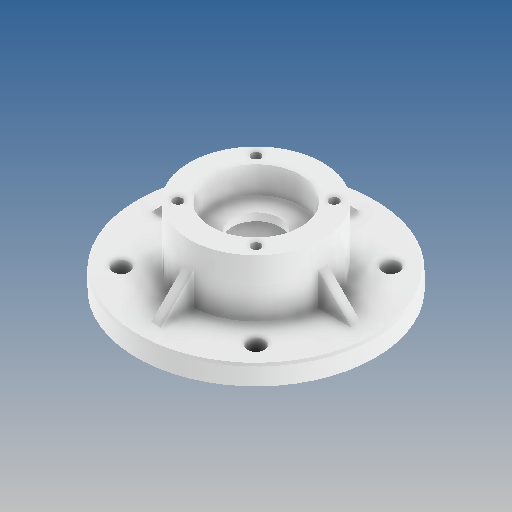
# Autodesk Inventor part: PWTR-0046
Saved by Autodesk Inventor 2021.1 (Build 251245000, 245)
## iProperties
Created: 2020-08-27
Part Number: PWTR-0046
Material: Aluminum 6061
Document SubType Name: Modeling
Designer: alid
Density: 2.7 g/cm^3
Appearance: Aluminum - Flat
Description: Transfer Case Connecting Plate
Author: alid
Revision Number: A
Autodesk Inventor part; units mm, degrees
ref_plane "YZ Plane" through (0, 0, 0) normal (1, 0, 0) x (0, 1, 0)
ref_plane "XZ Plane" through (0, 0, 0) normal (0, 1, 0) x (-1, 0, 0)
ref_plane "XY Plane" through (0, 0, 0) normal (0, 0, 1) x (1, 0, 0)
sketch "Sketch1" plane through (0, 0, 0) normal (0, 1, 0) x (-1, 0, 0)
  line L0 (0, 0) -> (0, 40)
  line L1 (0, 40) -> (-35, 40)
  line L2 (-35, 40) -> (-35, 10)
  line L3 (-35, 10) -> (-62.5, 10)
  line L4 (-62.5, 10) -> (-62.5, 0)
  line L5 (-62.5, 0) -> (0, 0)
  line L6 (-51.5, 11) -> (-36, 26.5)
  line L7 (-36, 40) -> (-36, 11) construction
  line L8 (-36, 11) -> (-72.5, 11) construction
  line L9 (-51.5, 11) -> (-52.5, 10) construction
  line L10 (0, 0) -> (0, -10)
  line L11 (0, -10) -> (-37.5, -10)
  line L12 (-37.5, -10) -> (-37.5, 0)
  dimension "d0" = 40
  dimension "d1" = 125
  dimension "d2" = 70
  dimension "d3" = 10
  dimension "d4" = 45
  dimension "d14" = 1
  dimension "d15" = 1
  dimension "d16" = 10
  dimension "d26" = 10
  dimension "d27" = 75
  constraints: 26 end point, 8 perpendicular, 4 point on line, 2 vertical, 1 collinear, 1 horizontal alignment, 1 parallel
  measures "d0" distance of L0.start L0.end
  measures "d1" diameter of L4 L0
  measures "d2" diameter of L2 L0
  measures "d3" distance between parallel lines of L5 L3
  measures "d4" angle of L3 L6
  measures "d14" distance between parallel lines of L3 L8
  measures "d15" distance between parallel lines of L2 L7
  measures "d16" distance from line of L4 L9.end
  measures "d26" distance of L0.start L10.end
  measures "d27" diameter of L12 L0
revolve "Revolution1" add sketch "Sketch1" angle 360 about axis through (0, 0, 0) along (0, 0, 1)
extrude "Rib1" add sketch "Sketch1" along normal mid plane 5 rib yes fills toward (-43.7146, 18.7146) open curves L6
sketch "Sketch3" plane through (0, 0, 40) normal (0, 0, 1) x (1, 0, 0)
  circle A0 centre (0, 0) radius 35 projected
  constraints: 1 coincident
hole "Hole2" at (0, 0, 40) direction (0, 0, -1) diameter 25 end through all counterbore diameter 47 counterbore depth 14
sketch "Sketch4" plane through (0, 0, 0) normal (0, 0, 1) x (1, 0, 0)
  circle A0 centre (0, 0) radius 50 construction
  line L0 (0, 0) -> (35.3553, 35.3553) construction
  line L1 (0, 0) -> (50, 0) construction
  dimension "d35" = 100
  dimension "d36" = 45
  constraints: 4 end point, 2 point on circle, 1 centre point, 1 coincident, 1 horizontal
  measures "d35" diameter of A0
  measures "d36" angle of L0 L1
hole "Hole3" at (35.3553, 35.3553, 0) direction (0, 0, 1) diameter 9 end through all clearance for "Hex Head Bolt" size "M8" standard "Ansi Metric M Profile"
pattern_circular "Circular Pattern1" count 4 over 360 about axis through (0, 0, -10) along (0, 0, 1) of "Rib1", "Hole3"
chamfer "Chamfer1" distance 1 angle 45 1 edges at (-62.5, 0, 10)
sketch "Sketch5" plane through (0, 0, 40) normal (0, 0, 1) x (1, 0, 0)
  circle A0 centre (0, 0) radius 29 construction
  line L0 (0, 0) -> (-20.5061, 20.5061) construction
  line L1 (0, 0) -> (0, 29) construction
  dimension "d47" = 58
  dimension "d48" = 45
  constraints: 4 end point, 2 point on circle, 1 centre point, 1 coincident, 1 vertical
  measures "d47" diameter of A0
  measures "d48" angle of L1 L0
hole "Hole4" at (-20.5061, 20.5061, 40) direction (0, 0, -1) diameter 4.917 depth 17.1 tip angle 118 thread size "M6x1" class "6H" standard "ISO Metric profile"
pattern_circular "Circular Pattern2" count 4 over 360 about axis through (0, 0, -10) along (0, 0, 1) of "Hole4"
sketch "Sketch6" plane through (0, 0, -10) normal (0, 0, -1) x (-1, 0, 0)
  circle A0 centre (0, 0) radius 37.5 projected
  constraints: 1 coincident
hole "Hole5" at (0, 0, -10) direction (0, 0, 1) diameter 47 depth 32 counterbore diameter 48 counterbore depth 8
thread "Thread1" size "M48x1.5" class "6H" standard "ISO Metric profile" full length
chamfer "Chamfer2" distance 0.5 angle 45 1 edges at (0, -24, -10)
equation "\"d15\" = d14"
body "Solid1"
